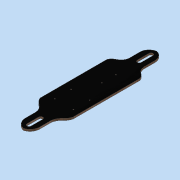
# Autodesk Inventor part: LongboardDeck
Saved by Autodesk Inventor 2015 SP1 (Build 190203100, 203)
## iProperties
Created: 2015-06-13
Part Number: LongboardDeck
Material: Wood (Birch)
Document SubType Name: Modeling
Designer: YOUR_NAME_HERE
Density: 0.55 g/cm^3
Appearance: Birch - Natural Polished
Author: YOUR_NAME_HERE
Autodesk Inventor part; units mm, degrees
sketch "Sketch1" plane through (0, 0, 0) normal (0, 1, 0) x (-1, 0, 0)
  line L0 (50.8, 457.2) -> (-50.8, 457.2) construction
  line L1 (-50.8, 457.2) -> (-50.8, 393.7) construction
  line L2 (-50.8, 393.7) -> (50.8, 393.7) construction
  line L3 (50.8, 393.7) -> (50.8, 457.2) construction
  line L4 (167.2348, 0) -> (-167.2348, 0) projected
  line L5 (0, -93.222) -> (0, 559.3318) projected
  arc A0 (50.8, 393.7) -> (0, 457.2) centre (-14.2875, 393.7) ccw
  arc A1 (0, 457.2) -> (-50.8, 393.7) centre (14.2875, 393.7) ccw
  line L6 (50.8, 393.7) -> (-50.8, 393.7) construction
  line L7 (-50.8, 393.7) -> (-50.8, 317.5)
  line L8 (-50.8, 317.5) -> (50.8, 317.5) construction
  line L9 (50.8, 317.5) -> (50.8, 393.7)
  line L10 (112.7125, 317.5) -> (-112.7125, 317.5) construction
  line L11 (-112.7125, 317.5) -> (-112.7125, 228.6) construction
  line L12 (-112.7125, 228.6) -> (112.7125, 228.6) construction
  line L13 (112.7125, 228.6) -> (112.7125, 317.5) construction
  line L14 (112.7125, 266.7) -> (-112.7125, 266.7) construction
  line L15 (82.55, 317.5) -> (82.55, 228.6) construction
  line L16 (-82.55, 317.5) -> (-82.55, 228.6) construction
  arc A2 (50.8, 317.5) -> (82.55, 266.7) centre (119.4534, 325.0865) ccw
  arc A3 (-82.55, 266.7) -> (-50.8, 317.5) centre (-119.4534, 325.0865) ccw
  arc A4 (112.7125, 228.6) -> (82.55, 266.7) centre (47.1527, 207.6878) ccw
  arc A5 (-82.55, 266.7) -> (-112.7125, 228.6) centre (-47.1527, 207.6878) ccw
  line L17 (112.7125, 228.6) -> (-112.7125, 228.6) construction
  line L18 (-112.7125, 228.6) -> (-112.7125, 0)
  line L19 (-112.7125, 0) -> (112.7125, 0)
  line L20 (112.7125, 0) -> (112.7125, 228.6)
  point P0 (0, 0)
  dimension "d0" = 50.8
  dimension "d1" = 63.5
  dimension "d2" = 76.2
  dimension "d3" = 88.9
  dimension "d4" = 225.425
  dimension "d5" = 50.8
  dimension "d6" = 165.1
  dimension "d7" = 69.0713
  dimension "d8" = 68.8143
  dimension "d9" = 457.2
  constraints: 38 end point, 12 point on circle, 11 point on line, 8 parallel, 6 centre point, 6 perpendicular, 4 horizontal, 4 symmetric about line, 2 collinear, 1 midpoint, 1 tangent, 1 vertical, 6 other
  measures "d0" distance between parallel lines of L5 L3
  measures "d1" distance between parallel lines of L2 L0
  measures "d2" distance of L8.end L2.end
  measures "d3" distance of L12.end L10.start
  measures "d4" distance of L11.end L12.end
  measures "d5" distance between parallel lines of L10 L14
  measures "d6" distance between parallel lines of L16 L15
  measures "d7" radius of A2
  measures "d8" radius of A4
  measures "d9" distance between parallel lines of L0 L19
extrude "Deck Base" add sketch "Sketch1" against normal blind 21.59
mirror "Deck Mirror" about plane through (-112.7125, 0, 0) normal (0, 0, -1) of "Deck Base"
sketch "Sketch3" plane through (0, 0, 0) normal (0, 1, 0) x (1, 0, 0)
  line L0 (0, -417.83) -> (0, -337.82) construction
  line L1 (13.97, -417.83) -> (13.97, -337.82)
  line L2 (-13.97, -337.82) -> (-13.97, -417.83)
  arc A0 (-13.97, -417.83) -> (13.97, -417.83) centre (0, -417.83) ccw
  arc A1 (13.97, -337.82) -> (-13.97, -337.82) centre (0, -337.82) ccw
  line L3 (50.8, -317.5) -> (50.8, -393.7) projected
  arc A2 (0, -457.2) -> (50.8, -393.7) centre (-14.2875, -393.7) ccw projected
  arc A3 (-50.8, -393.7) -> (0, -457.2) centre (14.2875, -393.7) ccw projected
  line L4 (-50.8, -393.7) -> (-50.8, -317.5) projected
  arc A4 (-50.8, -317.5) -> (-82.55, -266.7) centre (-119.4534, -325.0865) ccw projected
  arc A5 (-112.7125, -228.6) -> (-82.55, -266.7) centre (-47.1527, -207.6878) ccw projected
  line L5 (-112.7125, -228.6) -> (-112.7125, 228.6) projected
  arc A6 (-82.55, 266.7) -> (-112.7125, 228.6) centre (-47.1527, 207.6878) ccw projected
  arc A7 (-82.55, 266.7) -> (-50.8, 317.5) centre (-119.4534, 325.0865) ccw projected
  line L6 (-50.8, 317.5) -> (-50.8, 393.7) projected
  arc A8 (0, 457.2) -> (-50.8, 393.7) centre (14.2875, 393.7) ccw projected
  arc A9 (50.8, 393.7) -> (0, 457.2) centre (-14.2875, 393.7) ccw projected
  line L7 (50.8, 393.7) -> (50.8, 317.5) projected
  arc A10 (50.8, 317.5) -> (82.55, 266.7) centre (119.4534, 325.0865) ccw projected
  arc A11 (112.7125, 228.6) -> (82.55, 266.7) centre (47.1527, 207.6878) ccw projected
  line L8 (112.7125, 228.6) -> (112.7125, -228.6) projected
  arc A12 (82.55, -266.7) -> (112.7125, -228.6) centre (47.1527, -207.6878) ccw projected
  arc A13 (82.55, -266.7) -> (50.8, -317.5) centre (119.4534, -325.0865) ccw projected
  line L9 (0, 652.5538) -> (0, -652.5538) projected
  point P0 (0, 0)
  point P1 (0, -377.825)
  point P2 (0, -431.8)
  point P3 (0, -323.85)
  dimension "d16" = 25.4
  dimension "d17" = 27.94
  dimension "d18" = 107.95
  constraints: 8 end point, 6 point on circle, 4 tangent, 2 centre point, 1 collinear, 1 midpoint, 1 parallel, 1 point on line, 1 vertical
  measures "d16" distance of A2.start point (0, -431.8)
  measures "d17" distance between parallel lines of L1 L2
  measures "d18" distance of point (0, -431.8) point (0, -323.85)
extrude "Truck Hole" cut sketch "Sketch3" against normal through all contours A0 L9 A1 L1 | A0 L2 A1 L9
mirror "Truck Hole Mirror" about plane through (0, 0, 0) normal (0, 0, 1) of "Truck Hole"
sketch "Sketch2" plane through (0, 0, 0) normal (0, 0, 1) x (1, 0, 0)
  line L0 (-112.7125, -21.59) -> (-112.7125, 0) projected
  line L1 (-112.7125, 0) -> (112.7125, 0) projected
  line L2 (112.7125, 0) -> (112.7125, -21.59) projected
  line L3 (112.7125, -21.59) -> (-112.7125, -21.59) projected
  line L4 (-112.7125, -12.7) -> (112.7125, -12.7) construction
  line L5 (-112.7125, -8.89) -> (112.7125, -8.89) construction
  arc A0 (-112.7125, 0) -> (112.7125, 0) centre (0, 710.0717) ccw
  arc A1 (-112.7125, -12.7) -> (112.7125, -12.7) centre (0, 697.3717) ccw
  line L6 (-112.7125, 0) -> (-112.7125, -12.7)
  line L7 (112.7125, 0) -> (112.7125, -12.7)
  point P0 (0, 0)
  point P1 (0, -8.89)
  dimension "d12" = 12.7
  dimension "d13" = 8.89
  constraints: 8 end point, 5 point on circle, 4 point on line, 3 perpendicular, 2 centre point, 1 collinear, 1 midpoint, 1 tangent
  measures "d12" distance between parallel lines of L1 L4
  measures "d13" distance between parallel lines of L1 L5
extrude "Deck Curve" cut sketch "Sketch2" along normal through all both and the other way through all contours L0 A1 L3 | A1 L2 L3 | L1 A0
ref_plane "Top Plane" through (0, -8.89, 457.2) normal (0, 1, 0) x (-1, 0, 0)
ref_plane "Front Plane" through (0, -21.59, 457.2) normal (0, 0, 1) x (1, 0, 0)
ref_plane "Back Plane" through (0, -21.59, -457.2) normal (0, 0, 1) x (1, 0, 0)
sketch "Sketch5" plane through (0, -8.89, 457.2) normal (0, 1, 0) x (-1, 0, 0)
  line L0 (0, -1097.283) -> (0, 182.883) projected
  circle A0 centre (0, -538.48) radius 3.2639
  circle A1 centre (0, -635) radius 3.2639
  point P0 (0, -457.2)
  point P1 (0, -914.4)
  dimension "d23" = 6.5278
  dimension "d24" = 96.52
  dimension "d25" = 279.4
  constraints: 2 centre point, 2 point on line, 1 equal radius
  measures "d23" diameter of A0
  measures "d24" distance of A1.centre A0.centre
  measures "d25" distance of point (0, -914.4) A1.centre
extrude "Extrusion5" cut sketch "Sketch5" along normal through all both and the other way through all
sketch "Sketch6" plane through (0, 0, 0) normal (0, 1, 0) x (-1, 0, 0)
  circle A0 centre (63.627, 65.8876) radius 3.2639
  circle A1 centre (63.627, 177.8) radius 3.2639
  circle A2 centre (-63.627, 65.8876) radius 3.2639
  circle A3 centre (-63.627, 177.8) radius 3.2639
  line L0 (0, -640.083) -> (0, 640.083) projected
  line L1 (-157.8006, 457.2) -> (157.8006, 457.2) projected
  point P0 (0, 0)
  dimension "d28" = 111.9124
  dimension "d29" = 127.254
  dimension "d30" = 6.5278
  dimension "d31" = 279.4
  constraints: 4 centre point, 3 equal radius, 2 horizontal alignment, 2 vertical alignment, 1 symmetric about line
  measures "d28" distance of A1.centre A0.centre
  measures "d29" distance of A0.centre A2.centre
  measures "d30" diameter of A0
  measures "d31" distance from line of L1 A1.centre
extrude "Extrusion6" cut sketch "Sketch6" against normal through all
body "Solid1"
